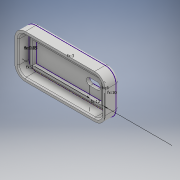
# Autodesk Inventor part: LED box top
Saved by Autodesk Inventor 2018.3 (Build 223284000, 284)
## iProperties
Created: 2019-07-19
Part Number: LED box top
Material: Generic
Document SubType Name: Modeling
Designer: uqspowe6
Density: 1 g/cm^3
Appearance: Default
Author: uqspowe6
Autodesk Inventor part; units mm, degrees
ref_plane "YZ Plane" through (0, 0, 0) normal (1, 0, 0) x (0, 1, 0)
ref_plane "XZ Plane" through (0, 0, 0) normal (0, 1, 0) x (-1, 0, 0)
ref_plane "XY Plane" through (0, 0, 0) normal (0, 0, 1) x (1, 0, 0)
derived "LED box.ipt"
sketch "Sketch3" plane through (-35.5, 40.5, -3) normal (0, 1, 0) x (1, 0, 0)
  line L0 (71, -31) -> (71, 0) construction
  line L1 (0, 0) -> (71, 0) construction
  line L2 (0, -31) -> (0, 0) construction
  line L3 (71, -31) -> (0, -31) construction
  line L4 (3, -25) -> (3, -6)
  line L5 (6, -3) -> (65, -3)
  line L6 (68, -6) -> (68, -25)
  line L7 (65, -28) -> (6, -28)
  arc A0 (3, -25) -> (6, -28) centre (6, -25) ccw
  arc A1 (6, -3) -> (3, -6) centre (6, -6) ccw
  arc A2 (68, -6) -> (65, -3) centre (65, -6) ccw
  arc A3 (65, -28) -> (68, -25) centre (65, -25) ccw
  line L8 (0, 0) -> (0, -31) construction
  line L9 (6, -31) -> (65, -31)
  line L10 (71, -25) -> (71, -6)
  line L11 (65, 0) -> (6, 0)
  line L12 (0, -6) -> (0, -25)
  arc A4 (0, -25) -> (6, -31) centre (6, -25) ccw
  arc A5 (6, 0) -> (0, -6) centre (6, -6) ccw
  arc A6 (71, -6) -> (65, 0) centre (65, -6) ccw
  arc A7 (65, -31) -> (71, -25) centre (65, -25) ccw
  point P0 (35.5, -3)
  point P1 (3, -28)
  point P2 (3, -3)
  point P3 (68, -3)
  point P4 (68, -28)
sketch "Sketch2" plane through (0, 0, 0) normal (0, 1, 0) x (-1, 0, 0)
  arc A0 (35.5, 22) -> (29.5, 28) centre (29.5, 22) ccw construction
  arc A1 (32.5, 22) -> (29.5, 25) centre (29.5, 22) ccw construction
  line L0 (32.5, 22) -> (32.5, 3) construction
  line L1 (-29.5, 25) -> (29.5, 25) construction
  line L2 (29.5, 0) -> (-29.5, 0) construction
  arc A2 (29.5, 0) -> (32.5, 3) centre (29.5, 3) ccw construction
  arc A3 (-29.5, 25) -> (-32.5, 22) centre (-29.5, 22) ccw construction
  arc A4 (-29.5, 28) -> (-35.5, 22) centre (-29.5, 22) ccw construction
  line L3 (-35.5, 22) -> (-35.5, 3) construction
  line L4 (-32.5, 3) -> (-32.5, 22) construction
  arc A5 (-32.5, 3) -> (-29.5, 0) centre (-29.5, 3) ccw construction
  arc A6 (-35.5, 3) -> (-29.5, -3) centre (-29.5, 3) ccw construction
  line L5 (35.5, 3) -> (35.5, 22) construction
  arc A7 (29.5, -3) -> (35.5, 3) centre (29.5, 3) ccw construction
  line L6 (29.5, 28) -> (-29.5, 28) construction
  line L7 (-29.5, -3) -> (29.5, -3) construction
  line L8 (32.45, 3) -> (32.45, 22)
  arc A8 (32.45, 22) -> (29.5, 24.95) centre (29.5, 22) ccw
  line L9 (29.5, 24.95) -> (-29.5, 24.95)
  arc A9 (-29.5, 24.95) -> (-32.45, 22) centre (-29.5, 22) ccw
  line L10 (-32.45, 22) -> (-32.45, 3)
  arc A10 (-32.45, 3) -> (-29.5, 0.05) centre (-29.5, 3) ccw
  line L11 (-29.5, 0.05) -> (29.5, 0.05)
  arc A11 (29.5, 0.05) -> (32.45, 3) centre (29.5, 3) ccw
  arc A12 (35.55, 22) -> (29.5, 28.05) centre (29.5, 22) ccw
  line L12 (29.5, 28.05) -> (-29.5, 28.05)
  arc A13 (-29.5, 28.05) -> (-35.55, 22) centre (-29.5, 22) ccw
  line L13 (-35.55, 22) -> (-35.55, 3)
  arc A14 (-35.55, 3) -> (-29.5, -3.05) centre (-29.5, 3) ccw
  line L14 (-29.5, -3.05) -> (29.5, -3.05)
  arc A15 (29.5, -3.05) -> (35.55, 3) centre (29.5, 3) ccw
  line L15 (35.55, 3) -> (35.55, 22)
  arc A16 (29.5, -6.05) -> (38.55, 3) centre (29.5, 3) ccw
  line L16 (29.5, -6.05) -> (-29.5, -6.05)
  arc A17 (-38.55, 3) -> (-29.5, -6.05) centre (-29.5, 3) ccw
  line L17 (-38.55, 3) -> (-38.55, 22)
  arc A18 (-29.5, 31.05) -> (-38.55, 22) centre (-29.5, 22) ccw
  line L18 (-29.5, 31.05) -> (29.5, 31.05)
  arc A19 (38.55, 22) -> (29.5, 31.05) centre (29.5, 22) ccw
  line L19 (38.55, 22) -> (38.55, 3)
  line L20 (-29.45, 21.95) -> (29.45, 21.95)
  line L21 (29.45, 21.95) -> (29.45, 3.05)
  line L22 (29.45, 3.05) -> (-29.45, 3.05)
  line L23 (-29.45, 3.05) -> (-29.45, 21.95)
  point P0 (0, 0)
  dimension "d1" = 0.05
  dimension "d2" = 0.05
  dimension "d3" = 3
  dimension "d27" = 3
  constraints: 32 end point, 24 point on circle, 12 centre point, 24 other
  measures "d1" distance between parallel lines of L0 L8
  measures "d2" distance between parallel lines of L5 L15
  measures "d3" radial gap between concentric circles of A15 A16
  measures "d27" distance between parallel lines of L9 L20
extrude "Extrusion1" add sketch "Sketch2" along normal blind 3 contours A11 L11 A10 L10 A9 L9 A8 L8 | L15 A15 L14 A14 L13 A13 L12 A12 | L16 A17 L17 A18 L18 A19 L19 A16 | L20 L21 L22 L23
extrude "Extrusion2" add sketch "Sketch2" against normal blind 3 contours A11 L11 A10 L10 A9 L9 A8 L8
extrude "Extrusion3" add sketch "Sketch2" against normal blind 9 contours L16 A17 L17 A18 L18 A19 L19 A16
chamfer "Chamfer1" distance 1 angle 45 16 edges at (-32.45, -3, 12.5) (-31.586, -3, 0.914) (0, -3, 0.05) (31.586, -3, 0.914) (32.45, -3, 12.5) (31.586, -3, 24.086) (0, -3, 24.95) (-31.586, -3, 24.086) (0, -9, 28.05) (33.778, -9, 26.278) (35.55, -9, 12.5) (33.778, -9, -1.278) (0, -9, -3.05) (-33.778, -9, -1.278) (-35.55, -9, 12.5) (-33.778, -9, 26.278)
fillet "Fillet1" radius 3 8 edges at (35.8993, 3, 28.3993) (38.55, 3, 12.5) (35.8993, 3, -3.3993) (0, 3, -6.05) (-35.8993, 3, -3.3993) (-38.55, 3, 12.5) (-35.8993, 3, 28.3993) (0, 3, 31.05)
sketch "Sketch4" plane through (0, 3, 0) normal (0, 1, 0) x (1, 0, 0)
  arc A0 (29.5, -28.05) -> (35.55, -22) centre (29.5, -22) ccw construction
  line L0 (35.55, -3) -> (35.55, -22) construction
  arc A1 (35.55, -3) -> (29.5, 3.05) centre (29.5, -3) ccw construction
  line L1 (-29.5, 3.05) -> (29.5, 3.05) construction
  arc A2 (-29.5, 3.05) -> (-35.55, -3) centre (-29.5, -3) ccw construction
  line L2 (-35.55, -22) -> (-35.55, -3) construction
  arc A3 (-35.55, -22) -> (-29.5, -28.05) centre (-29.5, -22) ccw construction
  line L3 (29.5, -28.05) -> (-29.5, -28.05) construction
  line L4 (13.55, -9.5) -> (25.55, -9.5)
  line L5 (25.55, -9.5) -> (25.55, -15.5)
  line L6 (25.55, -15.5) -> (13.55, -15.5)
  line L7 (13.55, -15.5) -> (13.55, -9.5)
  line L8 (35.55, -3) -> (35.55, -22) construction
  line L9 (35.55, -12.5) -> (-35.55, -12.5) construction
  line L10 (-35.55, -22) -> (-35.55, -3) construction
  point P0 (0, 0)
  dimension "d14" = 6
  dimension "d15" = 12
  dimension "d16" = 10
  constraints: 10 end point, 2 midpoint, 2 parallel, 1 horizontal, 1 perpendicular, 1 other
  measures "d14" distance of L4.end L5.end
  measures "d15" distance of L4.start L4.end
  measures "d16" distance between parallel lines of L8 L5
extrude "Extrusion4" cut sketch "Sketch4" against normal through all
fillet "Fillet2" radius 3 4 edges at (25.55, 1.5, 15.5) (25.55, 1.5, 9.5) (13.55, 1.5, 9.5) (13.55, 1.5, 15.5)
equation "\"d1\" = clearance"
equation "\"d2\" = clearance"
equation "\"d3\" = wall_t"
equation "\"d27\" = wall_t"
equation "\"d4\" = wall_t"
equation "\"d6\" = wall_t"
equation "\"d8\" = 3 * wall_t"
equation "\"d13\" = fillet_interior"
equation "\"d14\" = hole_h"
equation "\"d15\" = hole_w"
equation "\"d16\" = hole_offset"
equation "\"d28\" = hole_r"
equation "\"clearance\" = 0.05"
equation "\"hole_w\" = 12"
equation "\"hole_h\" = 6"
equation "\"hole_offset\" = 10"
equation "\"hole_r\" = 3"
equation "\"wall_t\" = 3"
equation "\"fillet_interior\" = 3"
body "Solid1"
